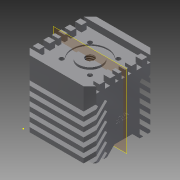
# Autodesk Inventor part: Heatsink
Saved by Autodesk Inventor 2015 (Build 190159000, 159)
## iProperties
Created: 2016-02-25
Part Number: Heatsink
Material: Aluminum 6061-AHC
Document SubType Name: Modeling
Designer: 672301
Density: 2.7 g/cm^3
Appearance: Anodized - Light Gray
Mass: 80.5123 g
Surface Area: 229.153 cm^2
Volume: 29.8194 cm^3
Author: 672301
Autodesk Inventor part; units mm, degrees
(part 1 of 2)
ref_plane "YZ Plane" through (0, 0, 0) normal (1, 0, 0) x (0, 1, 0)
ref_plane "XZ Plane" through (0, 0, 0) normal (0, 1, 0) x (-1, 0, 0)
sketch "Sketch1" plane through (0, 0, 0) normal (0, 1, 0) x (-1, 0, 0)
  line L0 (0, 0) -> (-40.005, 0)
  line L1 (-40.005, 0) -> (-40.005, -40.005)
  line L2 (-40.005, -40.005) -> (0, -40.005)
  line L3 (0, -40.005) -> (0, 0)
  dimension "d0" = 40.005
  dimension "d1" = 40.005
  constraints: 8 end point, 2 parallel, 1 horizontal, 1 perpendicular
  measures "d0" distance of L2.end L1.end
  measures "d1" distance of L0.end L1.end
extrude "Extrusion1" add sketch "Sketch1" along normal blind 40.005
sketch "Sketch2" plane through (0, 40.005, 0) normal (0, 1, 0) x (1, 0, 0)
  line L0 (0, 40.005) -> (0, 0) projected
  line L1 (0, 0) -> (40.005, 0) projected
  line L2 (0, 5.715) -> (40.005, 5.715)
  line L3 (0, 8.89) -> (40.005, 8.89)
  line L4 (0, 12.065) -> (40.005, 12.065)
  line L5 (0, 15.24) -> (40.005, 15.24)
  line L6 (40.005, 0) -> (40.005, 40.005) projected
  line L7 (0, 3.81) -> (40.005, 3.81)
  line L8 (0, 17.145) -> (40.005, 17.145)
  line L9 (0, 19.05) -> (40.005, 19.05)
  line L10 (0, 20.0025) -> (40.005, 20.0025) construction
  line L11 (0, 34.29) -> (40.005, 34.29)
  line L12 (0, 31.115) -> (40.005, 31.115)
  line L13 (0, 27.94) -> (40.005, 27.94)
  line L14 (0, 24.765) -> (40.005, 24.765)
  line L15 (0, 36.195) -> (40.005, 36.195)
  line L16 (0, 22.86) -> (40.005, 22.86)
  line L17 (0, 20.955) -> (40.005, 20.955)
  line L18 (0, 3.81) -> (0, 5.715)
  line L19 (40.005, 3.81) -> (40.005, 5.715)
  line L20 (0, 5.715) -> (0, 8.89)
  line L21 (0, 8.89) -> (0, 12.065)
  line L22 (0, 12.065) -> (0, 15.24)
  line L23 (0, 17.145) -> (0, 15.24)
  line L24 (0, 17.145) -> (0, 19.05)
  line L25 (0, 19.05) -> (0, 20.955)
  line L26 (0, 20.955) -> (0, 22.86)
  line L27 (0, 22.86) -> (0, 24.765)
  line L28 (0, 24.765) -> (0, 27.94)
  line L29 (0, 27.94) -> (0, 31.115)
  line L30 (0, 31.115) -> (0, 34.29)
  line L31 (0, 34.29) -> (0, 36.195)
  line L32 (0, 36.195) -> (0, 40.005)
  line L33 (40.005, 40.005) -> (40.005, 36.195)
  line L34 (40.005, 36.195) -> (40.005, 34.29)
  line L35 (40.005, 34.29) -> (40.005, 31.115)
  line L36 (40.005, 31.115) -> (40.005, 27.94)
  line L37 (40.005, 27.94) -> (40.005, 24.765)
  line L38 (40.005, 24.765) -> (40.005, 22.86)
  line L39 (40.005, 22.86) -> (40.005, 20.955)
  line L40 (40.005, 20.955) -> (40.005, 19.05)
  line L41 (40.005, 19.05) -> (40.005, 17.145)
  line L42 (40.005, 15.24) -> (40.005, 12.065)
  line L43 (40.005, 8.89) -> (40.005, 5.715)
  line L44 (40.005, 5.715) -> (40.005, 3.81)
  line L45 (40.005, 5.715) -> (40.005, 8.89)
  line L46 (0, 3.81) -> (0, 5.715)
  line L47 (40.005, 3.81) -> (40.005, 0)
  line L48 (0, 0) -> (0, 3.81)
  dimension "d5" = 5.715
  dimension "d6" = 8.89
  dimension "d7" = 12.065
  dimension "d8" = 15.24
  dimension "d9" = 3.81
  dimension "d10" = 17.145
  dimension "d11" = 19.05
  constraints: 92 end point, 17 collinear, 14 symmetric about line, 12 vertical, 4 horizontal, 4 point on line, 3 perpendicular, 2 parallel, 1 midpoint, 9 other
  measures "d5" distance between parallel lines of L1 L2
  measures "d6" distance between parallel lines of L1 L3
  measures "d7" distance between parallel lines of L1 L4
  measures "d8" distance between parallel lines of L1 L5
  measures "d9" distance between parallel lines of L1 L7
  measures "d10" distance between parallel lines of L1 L8
  measures "d11" distance between parallel lines of L1 L9
extrude "Extrusion2" cut sketch "Sketch2" against normal blind 3.81 contours L15 L6 L11 L0 | L12 L6 L13 L0 | L14 L6 L16 L0 | L17 L6 L9 L0 | L8 L6 L5 L0 | L4 L6 L3 L0 | L2 L6 L7 L0
sketch "Sketch3" plane through (0, 40.005, 0) normal (0, 1, 0) x (1, 0, 0)
  line L0 (0, 0) -> (0, 3.81)
  line L1 (0, 3.81) -> (3.81, 3.81)
  line L2 (40.005, 3.81) -> (0, 3.81) projected
  line L3 (40.005, 0) -> (40.005, 3.81)
  line L4 (40.005, 3.81) -> (36.195, 3.81)
  line L5 (0, 40.005) -> (0, 36.195)
  line L6 (0, 40.005) -> (0, 36.195) projected
  line L7 (0, 36.195) -> (3.81, 36.195)
  line L8 (0, 36.195) -> (40.005, 36.195) projected
  line L9 (40.005, 40.005) -> (40.005, 36.195)
  line L10 (40.005, 36.195) -> (40.005, 40.005) projected
  line L11 (40.005, 36.195) -> (36.195, 36.195)
  line L12 (3.81, 3.81) -> (36.195, 3.81)
  line L13 (36.195, 3.81) -> (36.195, 36.195)
  line L14 (36.195, 36.195) -> (3.81, 36.195)
  line L15 (3.81, 36.195) -> (3.81, 3.81)
  dimension "d14" = 3.81
  dimension "d15" = 3.81
  dimension "d16" = 3.81
  constraints: 24 end point, 4 equal length, 4 point on line, 2 vertical, 1 horizontal, 1 perpendicular
  measures "d14" distance of L0.start L0.end
  measures "d15" distance of L0.end L1.end
  measures "d16" distance of L2.start L4.end
extrude "Extrusion3" cut sketch "Sketch3" against normal up to surface (3.81 mm away)
sketch "Sketch4" plane through (0, 36.195, 0) normal (0, 1, 0) x (1, 0, 0)
  line L0 (40.005, 40.005) -> (0, 40.005) projected
  line L1 (0, 0) -> (40.005, 0) projected
  line L2 (0, 40.005) -> (0, 0) construction
  line L3 (0, 20.0025) -> (40.005, 20.0025) construction
  line L4 (40.005, 0) -> (40.005, 40.005) construction
  circle A0 centre (20.0025, 20.0025) radius 6.985
  circle A1 centre (20.0025, 20.0025) radius 10.668
  dimension "d19" = 13.97
  dimension "d20" = 21.336
  constraints: 3 midpoint, 2 centre point, 2 end point, 1 coincident
  measures "d19" diameter of A0
  measures "d20" diameter of A1
extrude "Extrusion4" cut sketch "Sketch4" against normal blind 0.762
sketch "Sketch5" plane through (0, 36.195, 0) normal (0, 1, 0) x (1, 0, 0)
  circle A0 centre (20.0025, 20.0025) radius 6.985 projected
  point P0 (0, 0)
extrude "Extrusion5" add sketch "Sketch5" along normal blind 0.508
hole "Hole1" at (20.0025, 36.703, -20.0025) direction (0, -1, 0) diameter 4.9784 end through all thread size "1/4-20 UNC" class "2B" standard "ANSI Unified Screw Threads"
sketch "Sketch6" plane through (0, 36.195, 0) normal (0, 1, 0) x (1, 0, 0)
  circle A0 centre (20.0025, 20.0025) radius 2.4892 projected
  circle A1 centre (20.0025, 20.0025) radius 6.985 projected
  line L0 (28.4861, 28.4861) -> (11.5189, 28.4861) construction
  line L1 (11.5189, 28.4861) -> (11.5189, 11.5189) construction
  line L2 (11.5189, 11.5189) -> (28.4861, 11.5189) construction
  line L3 (28.4861, 11.5189) -> (28.4861, 28.4861) construction
  line L4 (28.4861, 28.4861) -> (11.5189, 11.5189) construction
  line L5 (11.5189, 28.4861) -> (28.4861, 11.5189) construction
  point P0 (0, 0)
  dimension "d34" = 16.9672
  dimension "d35" = 16.9672
  constraints: 12 end point, 2 midpoint, 2 parallel, 1 horizontal, 1 perpendicular
  measures "d34" distance of L2.end L1.end
  measures "d35" distance of L1.end L0.end
hole "Hole2" at (28.4861, 36.195, -28.4861) at (11.5189, 36.195, -28.4861) at (11.5189, 36.195, -11.5189) at (28.4861, 36.195, -11.5189) direction (0, -1, 0) diameter 2.667 end through all
chamfer "Chamfer1" distance 3.81 angle 45 4 edges at (0, 20.0025, -40.005) (0, 20.0025, 0) (40.005, 20.0025, 0) (40.005, 20.0025, -40.005)
sketch "Sketch7" plane through (0, 0, 0) normal (0, -1, 0) x (1, 0, 0)
  line L0 (40.005, -3.81) -> (40.005, -14.605) construction
  line L1 (40.005, -3.81) -> (40.005, -36.195) projected
  line L2 (0, -36.195) -> (0, -3.81) projected
  line L3 (40.005, -14.605) -> (0, -14.605)
  line L4 (0, -14.605) -> (0, -25.4)
  line L5 (0, -25.4) -> (40.005, -25.4)
  line L6 (40.005, -25.4) -> (40.005, -14.605)
  point P0 (0, 0)
  dimension "d46" = 10.795
  dimension "d47" = 10.795
  constraints: 10 end point, 2 parallel, 2 point on line, 1 horizontal, 1 perpendicular
  measures "d46" distance of L0.start L0.end
  measures "d47" distance of L4.end L3.end
extrude "Extrusion6" cut sketch "Sketch7" against normal blind 4.445
sketch "Sketch8" plane through (0, 36.195, -5.715) normal (-1, 0, 0) x (0, 0, 1)
  line L0 (-8.89, -31.75) -> (-4.4778, -36.195)
  line L1 (-8.89, -36.195) -> (1.905, -36.195) projected
  line L2 (-19.685, -31.75) -> (-24.1046, -36.195)
  line L3 (-24.1046, -36.195) -> (-24.1046, 0) projected
  line L4 (-8.89, -31.75) -> (-8.89, -36.195)
  line L5 (-8.89, -31.75) -> (-8.89, -36.195) projected
  line L6 (-19.685, -31.75) -> (-19.685, -36.195)
  line L7 (-19.685, -36.195) -> (-19.685, -31.75) projected
  line L8 (-19.685, -36.195) -> (-24.1046, -36.195)
  line L9 (-30.48, -36.195) -> (-19.685, -36.195) projected
  point P0 (5.715, -36.195)
  constraints: 10 end point, 3 collinear, 2 point on line
extrude "Extrusion7" cut sketch "Sketch8" against normal through all contours L0 L1 L4
sketch "Sketch9" plane through (0, 36.195, -5.715) normal (-1, 0, 0) x (0, 0, 1)
  line L0 (-19.685, -31.75) -> (-24.1159, -36.195)
  line L1 (-30.48, -36.195) -> (-19.685, -36.195) projected
  line L2 (-19.685, -31.75) -> (-19.685, -36.195)
  line L3 (-19.685, -36.195) -> (-24.1159, -36.195)
  point P0 (5.715, -36.195)
  constraints: 6 end point, 1 perpendicular, 1 point on line, 1 vertical
extrude "Extrusion8" cut sketch "Sketch9" against normal through all
sketch "Sketch10" plane through (0, 4.445, 0) normal (0, -1, 0) x (1, 0, 0)
  circle A0 centre (20.0025, -20.0025) radius 2.4892 projected
  line L0 (36.195, -16.8275) -> (3.81, -16.8275)
  line L1 (3.81, -16.8275) -> (3.81, -23.1775)
  line L2 (3.81, -23.1775) -> (36.195, -23.1775)
  line L3 (36.195, -23.1775) -> (36.195, -16.8275)
  line L4 (36.195, -16.8275) -> (3.81, -23.1775) construction
  line L5 (3.81, -16.8275) -> (36.195, -23.1775) construction
  line L6 (40.005, -14.605) -> (40.005, -25.4) projected
  point P0 (0, 0)
  dimension "d54" = 32.385
  dimension "d55" = 6.35
  dimension "d56" = 3.81
  constraints: 12 end point, 2 midpoint, 2 parallel, 1 horizontal, 1 perpendicular
  measures "d54" distance of L2.end L1.end
  measures "d55" distance of L1.end L0.end
  measures "d56" distance between parallel lines of L6 L3
extrude "Extrusion9" cut sketch "Sketch10" against normal blind 16.51
sketch "Sketch12" plane through (36.195, 0, -40.005) normal (0, 0, -1) x (-1, 0, 0)
  point P0 (36.195, 0)
ref_plane "Work Plane1" through (3.81, 20.955, -20.0025) normal (0, 0, 1) x (1, 0, 0)
sketch "Sketch18" plane through (0, 36.195, -5.715) normal (-1, 0, 0) x (0, 0, 1)
  point P0 (5.715, -36.195)
sketch "Sketch19" plane through (0, 36.195, -5.715) normal (-1, 0, 0) x (0, 0, 1)
  point P0 (5.715, -36.195)
sketch "Sketch20" plane through (40.005, 36.195, -34.29) normal (1, 0, 0) x (0, 0, -1)
  line L0 (1.9052, -36.1976) -> (-4.4448, -36.1976)
  line L1 (1.9052, -36.1976) -> (5.7152, -36.1976)
  line L2 (5.7152, -36.1976) -> (5.7152, 3.8074)
  line L3 (5.7152, -36.1976) -> (-4.5592, -25.9231)
  line L4 (3.0212, -36.1976) -> (-4.5592, -28.6172)
  line L5 (0.3271, -36.1976) -> (-4.5592, -31.3113)
  line L6 (5.7152, -33.5035) -> (-4.5592, -23.2291)
  line L7 (-4.5592, -34.0054) -> (-2.367, -36.1976)
  line L8 (-4.5592, -20.535) -> (5.7152, -30.8094)
  line L9 (-4.5592, -17.8409) -> (5.7152, -28.1153)
  line L10 (-4.5592, -15.1468) -> (5.7152, -25.4213)
  line L11 (-4.5592, -12.4528) -> (5.7152, -22.7272)
  line L12 (-4.5592, -9.7587) -> (5.7152, -20.0331)
  line L13 (-4.5592, -7.0646) -> (5.7152, -17.339)
  line L14 (-3.2121, -5.7176) -> (5.7152, -14.645)
  line L15 (0.829, -7.0646) -> (5.7152, -11.9509)
  line L16 (2.176, -5.7176) -> (5.7152, -9.2568)
  line L17 (2.176, -5.7176) -> (0.829, -7.0646)
  line L18 (-3.2121, -5.7176) -> (5.7152, -5.7176)
  line L19 (-3.2121, -5.7176) -> (-4.5592, -7.0646)
  line L20 (-4.5592, -7.0646) -> (-4.5592, -36.0831)
  point P0 (-34.29, -36.195)
  dimension "d99" = 10.2744
  dimension "d85" = 45
  dimension "d86" = 1.905
  dimension "d87" = 3.81
  dimension "d88" = 1.905
  dimension "d89" = 1.905
  dimension "d90" = 1.905
  dimension "d91" = 1.905
  dimension "d92" = 1.905
  dimension "d93" = 1.905
  dimension "d94" = 1.905
  dimension "d95" = 1.905
  dimension "d96" = 1.905
  dimension "d97" = 1.905
  dimension "d98" = 1.905
  constraints: 38 end point, 12 parallel, 4 point on line, 2 horizontal, 2 perpendicular, 27 other
  measures "d85" angle of L0 L3
  measures "d86" distance between parallel lines of L4 L3
  measures "d87" distance between parallel lines of L3 L5
  measures "d88" distance between parallel lines of L3 L6
  measures "d89" distance between parallel lines of L5 L7
  measures "d90" distance between parallel lines of L6 L8
  measures "d91" distance between parallel lines of L8 L9
  measures "d92" distance between parallel lines of L9 L10
  measures "d93" distance between parallel lines of L10 L11
  measures "d94" distance between parallel lines of L11 L12
  measures "d95" distance between parallel lines of L12 L13
  measures "d96" distance between parallel lines of L13 L14
  measures "d97" distance between parallel lines of L14 L15
  measures "d98" distance between parallel lines of L15 L16
extrude "Extrusion14" cut sketch "Sketch20" against normal through all contours L0 L7 L20 L5 | L4 L20 L3 L1 | L6 L20 L8 L2 | L9 L20 L10 L2 | L11 L20 L12 L2 | L13 L19 L14 L2 | L15 L17 L16 L2
mirror "Mirror2" about plane through (3.81, 20.955, -20.0025) normal (0, 0, 1) of "Extrusion14"
sketch "Sketch21" plane through (0, 0, 0) normal (0, 1, 0) x (-1, 0, 0)
  point P0 (0, 0)
sketch "Sketch22" plane through (0, 0, 0) normal (0, -1, 0) x (1, 0, 0)
  arc A0 (11.3789, -10.1928) -> (11.6589, -10.1928) centre (11.5189, -11.5189) ccw projected
  arc A1 (28.3461, -10.1928) -> (28.6261, -10.1928) centre (28.4861, -11.5189) ccw projected
  circle A2 centre (20.0025, -20.0025) radius 2.4892 projected
  circle A3 centre (28.4861, -28.4861) radius 1.3335 projected
  circle A4 centre (11.5189, -28.4861) radius 1.3335 projected
  circle A5 centre (20.0025, -20.0025) radius 11.1125
  circle A6 centre (28.4861, -11.5189) radius 3.175
  circle A7 centre (11.5189, -11.5189) radius 3.175
  circle A8 centre (28.4861, -28.4861) radius 3.175
  circle A9 centre (11.5189, -28.4861) radius 3.175
  line L0 (38.8914, -2.6964) -> (1.1136, -2.6964) projected
  line L1 (0, -3.81) -> (1.1136, -2.6964) projected
  line L2 (0, -5.3905) -> (0, -3.81) projected
  line L3 (0, -5.3905) -> (40.005, -5.3905) projected
  line L4 (40.005, -3.81) -> (40.005, -5.3905) projected
  line L5 (38.8914, -2.6964) -> (40.005, -3.81) projected
  line L6 (40.005, -8.0846) -> (0, -8.0846) projected
  line L7 (0, -10.1928) -> (0, -8.0846) projected
  line L8 (0, -10.1928) -> (11.3789, -10.1928) projected
  arc A10 (11.6589, -10.1928) -> (11.3789, -10.1928) centre (11.5189, -11.5189) ccw projected
  line L9 (11.6589, -10.1928) -> (28.3461, -10.1928) projected
  arc A11 (28.6261, -10.1928) -> (28.3461, -10.1928) centre (28.4861, -11.5189) ccw projected
  line L10 (28.6261, -10.1928) -> (40.005, -10.1928) projected
  line L11 (40.005, -8.0846) -> (40.005, -10.1928) projected
  line L12 (0, -31.9204) -> (40.005, -31.9204) projected
  line L13 (40.005, -29.8309) -> (40.005, -31.9204) projected
  line L14 (40.005, -29.8309) -> (0, -29.8309) projected
  line L15 (0, -31.9204) -> (0, -29.8309) projected
  point P0 (0, 0)
  dimension "d103" = 22.225
  dimension "d105" = 6.35
  dimension "d106" = 6.35
  dimension "d107" = 6.35
  dimension "d108" = 6.35
  constraints: 5 centre point, 5 coincident
  measures "d103" diameter of A5
  measures "d105" diameter of A6
  measures "d106" diameter of A7
  measures "d107" diameter of A8
  measures "d108" diameter of A9
extrude "Extrusion15" cut sketch "Sketch22" against normal blind 31.115 contours A10 A0 A5 | A0 A5 A7 L8 | L8 A7 L9 A10 | A5 A0 | A0 A5 A7 | L9 A7 A5 A0 | A7 A5 L9 A6 A8 L14 A9 | A9 A5 A4 | A5 A4 A9 L14 | A5 L9 | L14 A9 | A6 L9 A1 A5 | A5 A1 A6 | A6 L10 A11 L9 | L14 A5 | A5 A1 | A1 A11 A5 | A5 A1 L10 A6 | A8 A5 A3 | A5 A3 A8 L14 | L14 A8
sketch "Sketch24" plane through (40.005, 4.445, -14.605) normal (1, 0, 0) x (0, 0, -1)
  line L0 (-4.2599, 13.3727) -> (14.146, 13.3727) construction
  line L1 (14.146, 13.3727) -> (14.146, 9.6523) construction
  line L2 (14.146, 9.6523) -> (-4.2599, 9.6523) construction
  line L3 (-4.2599, 9.6523) -> (-4.2599, 13.3727) construction
  spline S0 degree 2 poles (3.1149, 12.9571) (3.1149, 12.8527) (3.0303, 12.6848) (2.9593, 12.6378) knots 0 0 0 1 2 2 2
  spline S1 degree 2 poles (2.9593, 12.6378) (2.9013, 12.6014) (2.7821, 12.5767) (2.6895, 12.5767) knots 0 0 0 1 2 2 2
  line L4 (2.6895, 12.5767) -> (2.5141, 12.5767)
  line L5 (2.5141, 12.5767) -> (2.5141, 13.3387)
  line L6 (2.5141, 13.3387) -> (2.6876, 13.3387)
  spline S2 degree 2 poles (2.6876, 13.3387) (2.7951, 13.3387) (2.9173, 13.3066) (2.9606, 13.2782) knots 0 0 0 1 2 2 2
  spline S3 degree 2 poles (2.9606, 13.2782) (3.034, 13.2294) (3.1149, 13.0682) (3.1149, 12.9571) knots 0 0 0 1 2 2 2
  spline S4 degree 2 poles (3.0093, 12.9583) (3.0093, 13.046) (2.9513, 13.1701) (2.8939, 13.2053) knots 0 0 0 1 2 2 2
  spline S5 degree 2 poles (2.8939, 13.2053) (2.8531, 13.2294) (2.7611, 13.251) (2.6926, 13.251) knots 0 0 0 1 2 2 2
  line L7 (2.6926, 13.251) -> (2.6154, 13.251)
  line L8 (2.6154, 13.251) -> (2.6154, 12.6644)
  line L9 (2.6154, 12.6644) -> (2.6926, 12.6644)
  spline S6 degree 2 poles (2.6926, 12.6644) (2.7599, 12.6644) (2.8618, 12.686) (2.9031, 12.715) knots 0 0 0 1 2 2 2
  spline S7 degree 2 poles (2.9031, 12.715) (2.9562, 12.7508) (3.0093, 12.8694) (3.0093, 12.9583) knots 0 0 0 1 2 2 2
  spline S8 degree 2 poles (3.5361, 12.6372) (3.5243, 12.6286) (3.4848, 12.5977) (3.4663, 12.5884) knots 0 0 0 1 2 2 2
  spline S9 degree 2 poles (3.4663, 12.5884) (3.441, 12.5749) (3.3934, 12.5607) (3.3502, 12.5607) knots 0 0 0 1 2 2 2
  spline S10 degree 2 poles (3.3502, 12.5607) (3.315, 12.5607) (3.2514, 12.5872) (3.2273, 12.6113) knots 0 0 0 1 2 2 2
  spline S11 degree 2 poles (3.2273, 12.6113) (3.2045, 12.6348) (3.1767, 12.7039) (3.1767, 12.7422) knots 0 0 0 1 2 2 2
  spline S12 degree 2 poles (3.1767, 12.7422) (3.1767, 12.8015) (3.2267, 12.8855) (3.281, 12.9095) knots 0 0 0 1 2 2 2
  spline S13 degree 2 poles (3.281, 12.9095) (3.3292, 12.9318) (3.4601, 12.9485) (3.5361, 12.9528) knots 0 0 0 1 2 2 2
  line L10 (3.5361, 12.9528) -> (3.5361, 12.9713)
  spline S14 degree 2 poles (3.5361, 12.9713) (3.5361, 13.0046) (3.5157, 13.046) (3.4972, 13.0577) knots 0 0 0 1 2 2 2
  spline S15 degree 2 poles (3.4972, 13.0577) (3.4786, 13.0695) (3.4255, 13.0769) (3.3971, 13.0769) knots 0 0 0 1 2 2 2
  spline S16 degree 2 poles (3.3971, 13.0769) (3.3638, 13.0769) (3.2736, 13.0571) (3.2285, 13.038) knots 0 0 0 1 2 2 2
  line L11 (3.2285, 13.038) -> (3.223, 13.038)
  line L12 (3.223, 13.038) -> (3.223, 13.1362)
  spline S17 degree 2 poles (3.223, 13.1362) (3.2495, 13.1436) (3.349, 13.1621) (3.3977, 13.1621) knots 0 0 0 1 2 2 2
  spline S18 degree 2 poles (3.3977, 13.1621) (3.457, 13.1621) (3.5379, 13.1436) (3.57, 13.1195) knots 0 0 0 1 2 2 2
  spline S19 degree 2 poles (3.57, 13.1195) (3.6015, 13.096) (3.6324, 13.0213) (3.6324, 12.9676) knots 0 0 0 1 2 2 2
  line L13 (3.6324, 12.9676) -> (3.6324, 12.5767)
  line L14 (3.6324, 12.5767) -> (3.5361, 12.5767)
  line L15 (3.5361, 12.5767) -> (3.5361, 12.6372)
  line L16 (3.5361, 12.7175) -> (3.5361, 12.8762)
  spline S20 degree 2 poles (3.5361, 12.8762) (3.5015, 12.8731) (3.3971, 12.8626) (3.3644, 12.8527) knots 0 0 0 1 2 2 2
  spline S21 degree 2 poles (3.3644, 12.8527) (3.3261, 12.841) (3.2761, 12.7922) (3.2761, 12.749) knots 0 0 0 1 2 2 2
  spline S22 degree 2 poles (3.2761, 12.749) (3.2761, 12.6996) (3.3317, 12.6496) (3.3848, 12.6496) knots 0 0 0 1 2 2 2
  spline S23 degree 2 poles (3.3848, 12.6496) (3.4299, 12.6496) (3.504, 12.6885) (3.5361, 12.7175) knots 0 0 0 1 2 2 2
  line L17 (4.0708, 13.0454) -> (4.0659, 13.0454)
  spline S24 degree 2 poles (4.0659, 13.0454) (4.0548, 13.0485) (4.0307, 13.0497) (4.014, 13.0497) knots 0 0 0 1 2 2 2
  spline S25 degree 2 poles (4.014, 13.0497) (3.9751, 13.0497) (3.8985, 13.0158) (3.864, 12.9824) knots 0 0 0 1 2 2 2
  line L18 (3.864, 12.9824) -> (3.864, 12.5767)
  line L19 (3.864, 12.5767) -> (3.7676, 12.5767)
  line L20 (3.7676, 12.5767) -> (3.7676, 13.1485)
  line L21 (3.7676, 13.1485) -> (3.864, 13.1485)
  line L22 (3.864, 13.1485) -> (3.864, 13.0633)
  spline S26 degree 2 poles (3.864, 13.0633) (3.9164, 13.1102) (3.9949, 13.1485) (4.0319, 13.1485) knots 0 0 0 1 2 2 2
  spline S27 degree 2 poles (4.0319, 13.1485) (4.0467, 13.1485) (4.0616, 13.1473) (4.0708, 13.1454) knots 0 0 0 1 2 2 2
  line L23 (4.0708, 13.1454) -> (4.0708, 13.0454)
  spline S28 degree 2 poles (4.2999, 12.5631) (4.2425, 12.5631) (4.1431, 12.594) (4.1103, 12.6113) knots 0 0 0 1 2 2 2
  line L24 (4.1103, 12.6113) -> (4.1103, 12.7194)
  line L25 (4.1103, 12.7194) -> (4.1153, 12.7194)
  spline S29 degree 2 poles (4.1153, 12.7194) (4.1276, 12.7095) (4.161, 12.686) (4.1888, 12.673) knots 0 0 0 1 2 2 2
  spline S30 degree 2 poles (4.1888, 12.673) (4.2129, 12.6613) (4.2721, 12.644) (4.3036, 12.644) knots 0 0 0 1 2 2 2
  spline S31 degree 2 poles (4.3036, 12.644) (4.3265, 12.644) (4.379, 12.6545) (4.3913, 12.6632) knots 0 0 0 1 2 2 2
  spline S32 degree 2 poles (4.3913, 12.6632) (4.4092, 12.6749) (4.4253, 12.7014) (4.4253, 12.7286) knots 0 0 0 1 2 2 2
  spline S33 degree 2 poles (4.4253, 12.7286) (4.4253, 12.7626) (4.3882, 12.7978) (4.3407, 12.8095) knots 0 0 0 1 2 2 2
  spline S34 degree 2 poles (4.3407, 12.8095) (4.3221, 12.8138) (4.2629, 12.8262) (4.2376, 12.833) knots 0 0 0 1 2 2 2
  spline S35 degree 2 poles (4.2376, 12.833) (4.1721, 12.8521) (4.1128, 12.9312) (4.1128, 12.9874) knots 0 0 0 1 2 2 2
  spline S36 degree 2 poles (4.1128, 12.9874) (4.1128, 13.0652) (4.2295, 13.1621) (4.3259, 13.1621) knots 0 0 0 1 2 2 2
  spline S37 degree 2 poles (4.3259, 13.1621) (4.3734, 13.1621) (4.4697, 13.1386) (4.5025, 13.1207) knots 0 0 0 1 2 2 2
  line L26 (4.5025, 13.1207) -> (4.5025, 13.0176)
  line L27 (4.5025, 13.0176) -> (4.4975, 13.0176)
  spline S38 degree 2 poles (4.4975, 13.0176) (4.4605, 13.0473) (4.3703, 13.0812) (4.324, 13.0812) knots 0 0 0 1 2 2 2
  spline S39 degree 2 poles (4.324, 13.0812) (4.2765, 13.0812) (4.211, 13.0411) (4.211, 13.0009) knots 0 0 0 1 2 2 2
  spline S40 degree 2 poles (4.211, 13.0009) (4.211, 12.9645) (4.2499, 12.9293) (4.2931, 12.9182) knots 0 0 0 1 2 2 2
  spline S41 degree 2 poles (4.2931, 12.9182) (4.3141, 12.9126) (4.3672, 12.9015) (4.3962, 12.8947) knots 0 0 0 1 2 2 2
  spline S42 degree 2 poles (4.3962, 12.8947) (4.4592, 12.8787) (4.5235, 12.8052) (4.5235, 12.7416) knots 0 0 0 1 2 2 2
  spline S43 degree 2 poles (4.5235, 12.7416) (4.5235, 12.7045) (4.4944, 12.6391) (4.466, 12.615) knots 0 0 0 1 2 2 2
  spline S44 degree 2 poles (4.466, 12.615) (4.4358, 12.5897) (4.3586, 12.5631) (4.2999, 12.5631) knots 0 0 0 1 2 2 2
  line L28 (5.0619, 12.5767) -> (4.9656, 12.5767)
  line L29 (4.9656, 12.5767) -> (4.9656, 12.9028)
  spline S45 degree 2 poles (4.9656, 12.9028) (4.9656, 12.9423) (4.9582, 13.0102) (4.9471, 13.0306) knots 0 0 0 1 2 2 2
  spline S46 degree 2 poles (4.9471, 13.0306) (4.9353, 13.0522) (4.8933, 13.0732) (4.8575, 13.0732) knots 0 0 0 1 2 2 2
  spline S47 degree 2 poles (4.8575, 13.0732) (4.8217, 13.0732) (4.7458, 13.0349) (4.7093, 13.004) knots 0 0 0 1 2 2 2
  line L30 (4.7093, 13.004) -> (4.7093, 12.5767)
  line L31 (4.7093, 12.5767) -> (4.613, 12.5767)
  line L32 (4.613, 12.5767) -> (4.613, 13.3727)
  line L33 (4.613, 13.3727) -> (4.7093, 13.3727)
  line L34 (4.7093, 13.3727) -> (4.7093, 13.0849)
  spline S48 degree 2 poles (4.7093, 13.0849) (4.7525, 13.1238) (4.8359, 13.1646) (4.8828, 13.1646) knots 0 0 0 1 2 2 2
  spline S49 degree 2 poles (4.8828, 13.1646) (4.9668, 13.1646) (5.0619, 13.0534) (5.0619, 12.9478) knots 0 0 0 1 2 2 2
  line L35 (5.0619, 12.9478) -> (5.0619, 12.5767)
  line L36 (5.2953, 12.5767) -> (5.199, 12.5767)
  line L37 (5.199, 12.5767) -> (5.199, 13.1485)
  line L38 (5.199, 13.1485) -> (5.2953, 13.1485)
  line L39 (5.2953, 13.1485) -> (5.2953, 12.5767)
  line L40 (5.3021, 13.2436) -> (5.1928, 13.2436)
  line L41 (5.1928, 13.2436) -> (5.1928, 13.3437)
  line L42 (5.1928, 13.3437) -> (5.3021, 13.3437)
  line L43 (5.3021, 13.3437) -> (5.3021, 13.2436)
  line L44 (5.5349, 12.5767) -> (5.4386, 12.5767)
  line L45 (5.4386, 12.5767) -> (5.4386, 13.3727)
  line L46 (5.4386, 13.3727) -> (5.5349, 13.3727)
  line L47 (5.5349, 13.3727) -> (5.5349, 12.5767)
  spline S50 degree 2 poles (6.3087, 12.5631) (6.2346, 12.5631) (6.1092, 12.6131) (6.0635, 12.6632) knots 0 0 0 1 2 2 2
  spline S51 degree 2 poles (6.0635, 12.6632) (6.0178, 12.7126) (5.9678, 12.8608) (5.9678, 12.9571) knots 0 0 0 1 2 2 2
  spline S52 degree 2 poles (5.9678, 12.9571) (5.9678, 13.0528) (6.0166, 13.1948) (6.0629, 13.2473) knots 0 0 0 1 2 2 2
  spline S53 degree 2 poles (6.0629, 13.2473) (6.1086, 13.2986) (6.2333, 13.3523) (6.3105, 13.3523) knots 0 0 0 1 2 2 2
  spline S54 degree 2 poles (6.3105, 13.3523) (6.3488, 13.3523) (6.4161, 13.3412) (6.4445, 13.3325) knots 0 0 0 1 2 2 2
  spline S55 degree 2 poles (6.4445, 13.3325) (6.4692, 13.3245) (6.5205, 13.3017) (6.5458, 13.2881) knots 0 0 0 1 2 2 2
  line L48 (6.5458, 13.2881) -> (6.5458, 13.1658)
  line L49 (6.5458, 13.1658) -> (6.5378, 13.1658)
  spline S56 degree 2 poles (6.5378, 13.1658) (6.5242, 13.1782) (6.4822, 13.2127) (6.4519, 13.2294) knots 0 0 0 1 2 2 2
  spline S57 degree 2 poles (6.4519, 13.2294) (6.4229, 13.2455) (6.3544, 13.2658) (6.3099, 13.2658) knots 0 0 0 1 2 2 2
  spline S58 degree 2 poles (6.3099, 13.2658) (6.2611, 13.2658) (6.174, 13.2257) (6.1413, 13.1874) knots 0 0 0 1 2 2 2
  spline S59 degree 2 poles (6.1413, 13.1874) (6.1092, 13.1485) (6.0734, 13.0306) (6.0734, 12.9571) knots 0 0 0 1 2 2 2
  spline S60 degree 2 poles (6.0734, 12.9571) (6.0734, 12.8787) (6.1111, 12.7657) (6.1438, 12.7268) knots 0 0 0 1 2 2 2
  spline S61 degree 2 poles (6.1438, 12.7268) (6.1759, 12.6891) (6.2617, 12.6508) (6.3099, 12.6508) knots 0 0 0 1 2 2 2
  spline S62 degree 2 poles (6.3099, 12.6508) (6.3537, 12.6508) (6.4285, 12.6724) (6.4575, 12.6885) knots 0 0 0 1 2 2 2
  spline S63 degree 2 poles (6.4575, 12.6885) (6.4853, 12.7045) (6.5266, 12.7379) (6.5384, 12.7496) knots 0 0 0 1 2 2 2
  line L50 (6.5384, 12.7496) -> (6.5458, 12.7496)
  line L51 (6.5458, 12.7496) -> (6.5458, 12.6286)
  spline S64 degree 2 poles (6.5458, 12.6286) (6.5205, 12.6169) (6.476, 12.5952) (6.4445, 12.5854) knots 0 0 0 1 2 2 2
  spline S65 degree 2 poles (6.4445, 12.5854) (6.4112, 12.5742) (6.3544, 12.5631) (6.3087, 12.5631) knots 0 0 0 1 2 2 2
  spline S66 degree 2 poles (7.1028, 12.8626) (7.1028, 12.7181) (6.9638, 12.5607) (6.8477, 12.5607) knots 0 0 0 1 2 2 2
  spline S67 degree 2 poles (6.8477, 12.5607) (6.7286, 12.5607) (6.5921, 12.7231) (6.5921, 12.8626) knots 0 0 0 1 2 2 2
  spline S68 degree 2 poles (6.5921, 12.8626) (6.5921, 13.0059) (6.7329, 13.1646) (6.8477, 13.1646) knots 0 0 0 1 2 2 2
  spline S69 degree 2 poles (6.8477, 13.1646) (6.9638, 13.1646) (7.1028, 13.0065) (7.1028, 12.8626) knots 0 0 0 1 2 2 2
  spline S70 degree 2 poles (7.0034, 12.8626) (7.0034, 12.9738) (6.9225, 13.0818) (6.8477, 13.0818) knots 0 0 0 1 2 2 2
  spline S71 degree 2 poles (6.8477, 13.0818) (6.773, 13.0818) (6.6915, 12.9738) (6.6915, 12.8626) knots 0 0 0 1 2 2 2
  spline S72 degree 2 poles (6.6915, 12.8626) (6.6915, 12.7546) (6.773, 12.6434) (6.8477, 12.6434) knots 0 0 0 1 2 2 2
  spline S73 degree 2 poles (6.8477, 12.6434) (6.9218, 12.6434) (7.0034, 12.7527) (7.0034, 12.8626) knots 0 0 0 1 2 2 2
  line L52 (7.351, 12.5767) -> (7.2287, 12.5767)
  line L53 (7.2287, 12.5767) -> (7.2287, 12.7224)
  line L54 (7.2287, 12.7224) -> (7.351, 12.7224)
  line L55 (7.351, 12.7224) -> (7.351, 12.5767)
  spline S74 degree 2 poles (1.452, 11.8544) (1.452, 11.805) (1.4168, 11.7161) (1.3853, 11.6852) knots 0 0 0 1 2 2 2
  spline S75 degree 2 poles (1.3853, 11.6852) (1.3458, 11.6463) (1.239, 11.6062) (1.1574, 11.6062) knots 0 0 0 1 2 2 2
  line L56 (1.1574, 11.6062) -> (1.0716, 11.6062)
  line L57 (1.0716, 11.6062) -> (1.0716, 11.3221)
  line L58 (1.0716, 11.3221) -> (0.9703, 11.3221)
  line L59 (0.9703, 11.3221) -> (0.9703, 12.0841)
  line L60 (0.9703, 12.0841) -> (1.1618, 12.0841)
  spline S76 degree 2 poles (1.1618, 12.0841) (1.2297, 12.0841) (1.3248, 12.0619) (1.3612, 12.0366) knots 0 0 0 1 2 2 2
  spline S77 degree 2 poles (1.3612, 12.0366) (1.4038, 12.0075) (1.452, 11.918) (1.452, 11.8544) knots 0 0 0 1 2 2 2
  spline S78 degree 2 poles (1.3464, 11.8513) (1.3464, 11.8908) (1.3192, 11.9489) (1.2914, 11.9674) knots 0 0 0 1 2 2 2
  spline S79 degree 2 poles (1.2914, 11.9674) (1.2674, 11.9834) (1.2031, 11.9964) (1.1556, 11.9964) knots 0 0 0 1 2 2 2
  line L61 (1.1556, 11.9964) -> (1.0716, 11.9964)
  line L62 (1.0716, 11.9964) -> (1.0716, 11.6926)
  line L63 (1.0716, 11.6926) -> (1.1408, 11.6926)
  spline S80 degree 2 poles (1.1408, 11.6926) (1.2025, 11.6926) (1.2785, 11.7124) (1.3032, 11.7383) knots 0 0 0 1 2 2 2
  spline S81 degree 2 poles (1.3032, 11.7383) (1.326, 11.7611) (1.3464, 11.8149) (1.3464, 11.8513) knots 0 0 0 1 2 2 2
  spline S82 degree 2 poles (1.8595, 11.3826) (1.8478, 11.374) (1.8083, 11.3431) (1.7898, 11.3338) knots 0 0 0 1 2 2 2
  spline S83 degree 2 poles (1.7898, 11.3338) (1.7644, 11.3202) (1.7169, 11.306) (1.6737, 11.306) knots 0 0 0 1 2 2 2
  spline S84 degree 2 poles (1.6737, 11.306) (1.6385, 11.306) (1.5749, 11.3326) (1.5508, 11.3567) knots 0 0 0 1 2 2 2
  spline S85 degree 2 poles (1.5508, 11.3567) (1.5279, 11.3801) (1.5002, 11.4493) (1.5002, 11.4876) knots 0 0 0 1 2 2 2
  spline S86 degree 2 poles (1.5002, 11.4876) (1.5002, 11.5469) (1.5502, 11.6309) (1.6045, 11.6549) knots 0 0 0 1 2 2 2
  spline S87 degree 2 poles (1.6045, 11.6549) (1.6527, 11.6772) (1.7836, 11.6938) (1.8595, 11.6982) knots 0 0 0 1 2 2 2
  line L64 (1.8595, 11.6982) -> (1.8595, 11.7167)
  spline S88 degree 2 poles (1.8595, 11.7167) (1.8595, 11.75) (1.8392, 11.7914) (1.8206, 11.8031) knots 0 0 0 1 2 2 2
  spline S89 degree 2 poles (1.8206, 11.8031) (1.8021, 11.8149) (1.749, 11.8223) (1.7206, 11.8223) knots 0 0 0 1 2 2 2
  spline S90 degree 2 poles (1.7206, 11.8223) (1.6873, 11.8223) (1.5971, 11.8025) (1.552, 11.7834) knots 0 0 0 1 2 2 2
  line L65 (1.552, 11.7834) -> (1.5465, 11.7834)
  line L66 (1.5465, 11.7834) -> (1.5465, 11.8816)
  spline S91 degree 2 poles (1.5465, 11.8816) (1.573, 11.889) (1.6724, 11.9075) (1.7212, 11.9075) knots 0 0 0 1 2 2 2
  spline S92 degree 2 poles (1.7212, 11.9075) (1.7805, 11.9075) (1.8614, 11.889) (1.8935, 11.8649) knots 0 0 0 1 2 2 2
  spline S93 degree 2 poles (1.8935, 11.8649) (1.925, 11.8414) (1.9559, 11.7667) (1.9559, 11.713) knots 0 0 0 1 2 2 2
  line L67 (1.9559, 11.713) -> (1.9559, 11.3221)
  line L68 (1.9559, 11.3221) -> (1.8595, 11.3221)
  line L69 (1.8595, 11.3221) -> (1.8595, 11.3826)
  line L70 (1.8595, 11.4629) -> (1.8595, 11.6216)
  spline S94 degree 2 poles (1.8595, 11.6216) (1.825, 11.6185) (1.7206, 11.608) (1.6879, 11.5981) knots 0 0 0 1 2 2 2
  spline S95 degree 2 poles (1.6879, 11.5981) (1.6496, 11.5864) (1.5996, 11.5376) (1.5996, 11.4944) knots 0 0 0 1 2 2 2
  spline S96 degree 2 poles (1.5996, 11.4944) (1.5996, 11.445) (1.6551, 11.395) (1.7083, 11.395) knots 0 0 0 1 2 2 2
  spline S97 degree 2 poles (1.7083, 11.395) (1.7533, 11.395) (1.8274, 11.4339) (1.8595, 11.4629) knots 0 0 0 1 2 2 2
  line L71 (2.3943, 11.7908) -> (2.3894, 11.7908)
  spline S98 degree 2 poles (2.3894, 11.7908) (2.3782, 11.7939) (2.3542, 11.7951) (2.3375, 11.7951) knots 0 0 0 1 2 2 2
  spline S99 degree 2 poles (2.3375, 11.7951) (2.2986, 11.7951) (2.222, 11.7611) (2.1874, 11.7278) knots 0 0 0 1 2 2 2
  line L72 (2.1874, 11.7278) -> (2.1874, 11.3221)
  line L73 (2.1874, 11.3221) -> (2.0911, 11.3221)
  line L74 (2.0911, 11.3221) -> (2.0911, 11.8939)
  line L75 (2.0911, 11.8939) -> (2.1874, 11.8939)
  line L76 (2.1874, 11.8939) -> (2.1874, 11.8087)
  spline S100 degree 2 poles (2.1874, 11.8087) (2.2399, 11.8556) (2.3183, 11.8939) (2.3554, 11.8939) knots 0 0 0 1 2 2 2
  spline S101 degree 2 poles (2.3554, 11.8939) (2.3702, 11.8939) (2.385, 11.8927) (2.3943, 11.8908) knots 0 0 0 1 2 2 2
  line L77 (2.3943, 11.8908) -> (2.3943, 11.7908)
  spline S102 degree 2 poles (2.6419, 11.311) (2.5635, 11.311) (2.4752, 11.4005) (2.4752, 11.4975) knots 0 0 0 1 2 2 2
  line L78 (2.4752, 11.4975) -> (2.4752, 11.8143)
  line L79 (2.4752, 11.8143) -> (2.4104, 11.8143)
  line L80 (2.4104, 11.8143) -> (2.4104, 11.8939)
  line L81 (2.4104, 11.8939) -> (2.4752, 11.8939)
  line L82 (2.4752, 11.8939) -> (2.4752, 12.0582)
  line L83 (2.4752, 12.0582) -> (2.5715, 12.0582)
  line L84 (2.5715, 12.0582) -> (2.5715, 11.8939)
  line L85 (2.5715, 11.8939) -> (2.7487, 11.8939)
  line L86 (2.7487, 11.8939) -> (2.7487, 11.8143)
  line L87 (2.7487, 11.8143) -> (2.5715, 11.8143)
  line L88 (2.5715, 11.8143) -> (2.5715, 11.5419)
  spline S103 degree 2 poles (2.5715, 11.5419) (2.5715, 11.4987) (2.5746, 11.4512) (2.5851, 11.4308) knots 0 0 0 1 2 2 2
  spline S104 degree 2 poles (2.5851, 11.4308) (2.5938, 11.4129) (2.6327, 11.395) (2.666, 11.395) knots 0 0 0 1 2 2 2
  spline S105 degree 2 poles (2.666, 11.395) (2.6895, 11.395) (2.7333, 11.4092) (2.7432, 11.4135) knots 0 0 0 1 2 2 2
  line L89 (2.7432, 11.4135) -> (2.7487, 11.4135)
  line L90 (2.7487, 11.4135) -> (2.7487, 11.327)
  spline S106 degree 2 poles (2.7487, 11.327) (2.7216, 11.3196) (2.666, 11.311) (2.6419, 11.311) knots 0 0 0 1 2 2 2
  line L91 (3.6997, 11.3221) -> (3.5861, 11.3221)
  line L92 (3.5861, 11.3221) -> (3.2489, 11.9791)
  line L93 (3.2489, 11.9791) -> (3.2489, 11.3221)
  line L94 (3.2489, 11.3221) -> (3.1544, 11.3221)
  line L95 (3.1544, 11.3221) -> (3.1544, 12.0841)
  line L96 (3.1544, 12.0841) -> (3.2983, 12.0841)
  line L97 (3.2983, 12.0841) -> (3.6052, 11.4808)
  line L98 (3.6052, 11.4808) -> (3.6052, 12.0841)
  line L99 (3.6052, 12.0841) -> (3.6997, 12.0841)
  line L100 (3.6997, 12.0841) -> (3.6997, 11.3221)
  spline S107 degree 2 poles (4.3166, 11.608) (4.3166, 11.4635) (4.1777, 11.306) (4.0616, 11.306) knots 0 0 0 1 2 2 2
  spline S108 degree 2 poles (4.0616, 11.306) (3.9424, 11.306) (3.8059, 11.4684) (3.8059, 11.608) knots 0 0 0 1 2 2 2
  spline S109 degree 2 poles (3.8059, 11.608) (3.8059, 11.7513) (3.9467, 11.91) (4.0616, 11.91) knots 0 0 0 1 2 2 2
  spline S110 degree 2 poles (4.0616, 11.91) (4.1777, 11.91) (4.3166, 11.7519) (4.3166, 11.608) knots 0 0 0 1 2 2 2
  spline S111 degree 2 poles (4.2172, 11.608) (4.2172, 11.7192) (4.1363, 11.8272) (4.0616, 11.8272) knots 0 0 0 1 2 2 2
  spline S112 degree 2 poles (4.0616, 11.8272) (3.9868, 11.8272) (3.9053, 11.7192) (3.9053, 11.608) knots 0 0 0 1 2 2 2
  spline S113 degree 2 poles (3.9053, 11.608) (3.9053, 11.4999) (3.9868, 11.3888) (4.0616, 11.3888) knots 0 0 0 1 2 2 2
  spline S114 degree 2 poles (4.0616, 11.3888) (4.1357, 11.3888) (4.2172, 11.4981) (4.2172, 11.608) knots 0 0 0 1 2 2 2
  line L101 (4.5648, 11.3221) -> (4.4426, 11.3221)
  line L102 (4.4426, 11.3221) -> (4.4426, 11.4678)
  line L103 (4.4426, 11.4678) -> (4.5648, 11.4678)
  line L104 (4.5648, 11.4678) -> (4.5648, 11.3221)
  line L105 (5.5158, 11.3221) -> (5.0459, 11.3221)
  line L106 (5.0459, 11.3221) -> (5.0459, 11.4302)
  spline S115 degree 2 poles (5.0459, 11.4302) (5.0965, 11.4777) (5.1867, 11.566) (5.2299, 11.6136) knots 0 0 0 1 2 2 2
  spline S116 degree 2 poles (5.2299, 11.6136) (5.3169, 11.7093) (5.3806, 11.8241) (5.3806, 11.8853) knots 0 0 0 1 2 2 2
  spline S117 degree 2 poles (5.3806, 11.8853) (5.3806, 11.9174) (5.3608, 11.9655) (5.3429, 11.981) knots 0 0 0 1 2 2 2
  spline S118 degree 2 poles (5.3429, 11.981) (5.325, 11.9964) (5.278, 12.0119) (5.2496, 12.0119) knots 0 0 0 1 2 2 2
  spline S119 degree 2 poles (5.2496, 12.0119) (5.2225, 12.0119) (5.1669, 11.9983) (5.1416, 11.9878) knots 0 0 0 1 2 2 2
  spline S120 degree 2 poles (5.1416, 11.9878) (5.12, 11.9791) (5.0798, 11.9544) (5.0675, 11.9458) knots 0 0 0 1 2 2 2
  line L107 (5.0675, 11.9458) -> (5.0619, 11.9458)
  line L108 (5.0619, 11.9458) -> (5.0619, 12.0545)
  spline S121 degree 2 poles (5.0619, 12.0545) (5.0934, 12.0699) (5.2064, 12.1002) (5.2571, 12.1002) knots 0 0 0 1 2 2 2
  spline S122 degree 2 poles (5.2571, 12.1002) (5.3639, 12.1002) (5.4843, 11.9872) (5.4843, 11.8908) knots 0 0 0 1 2 2 2
  spline S123 degree 2 poles (5.4843, 11.8908) (5.4843, 11.8457) (5.4633, 11.7704) (5.4448, 11.7383) knots 0 0 0 1 2 2 2
  spline S124 degree 2 poles (5.4448, 11.7383) (5.4262, 11.705) (5.3725, 11.6395) (5.3429, 11.608) knots 0 0 0 1 2 2 2
  spline S125 degree 2 poles (5.3429, 11.608) (5.2947, 11.5555) (5.1768, 11.4431) (5.1416, 11.4104) knots 0 0 0 1 2 2 2
  line L109 (5.1416, 11.4104) -> (5.5158, 11.4104)
  line L110 (5.5158, 11.4104) -> (5.5158, 11.3221)
  line L111 (6.108, 11.5839) -> (6.0172, 11.5839)
  line L112 (6.0172, 11.5839) -> (6.0172, 11.3221)
  line L113 (6.0172, 11.3221) -> (5.919, 11.3221)
  line L114 (5.919, 11.3221) -> (5.919, 11.5839)
  line L115 (5.919, 11.5839) -> (5.5825, 11.5839)
  line L116 (5.5825, 11.5839) -> (5.5825, 11.6914)
  line L117 (5.5825, 11.6914) -> (5.9233, 12.0841)
  line L118 (5.9233, 12.0841) -> (6.0172, 12.0841)
  line L119 (6.0172, 12.0841) -> (6.0172, 11.6661)
  line L120 (6.0172, 11.6661) -> (6.108, 11.6661)
  line L121 (6.108, 11.6661) -> (6.108, 11.5839)
  line L122 (5.919, 11.6661) -> (5.919, 11.9637)
  line L123 (5.919, 11.9637) -> (5.6628, 11.6661)
  line L124 (5.6628, 11.6661) -> (5.919, 11.6661)
  spline S126 degree 2 poles (6.6514, 11.5642) (6.6514, 11.5092) (6.6162, 11.4153) (6.5841, 11.3808) knots 0 0 0 1 2 2 2
  spline S127 degree 2 poles (6.5841, 11.3808) (6.552, 11.3462) (6.4562, 11.306) (6.397, 11.306) knots 0 0 0 1 2 2 2
  spline S128 degree 2 poles (6.397, 11.306) (6.3426, 11.306) (6.2364, 11.3301) (6.1975, 11.3493) knots 0 0 0 1 2 2 2
  line L125 (6.1975, 11.3493) -> (6.1975, 11.4573)
  line L126 (6.1975, 11.4573) -> (6.2049, 11.4573)
  spline S129 degree 2 poles (6.2049, 11.4573) (6.2167, 11.4487) (6.2605, 11.4265) (6.287, 11.4166) knots 0 0 0 1 2 2 2
  spline S130 degree 2 poles (6.287, 11.4166) (6.3173, 11.4061) (6.3673, 11.3943) (6.3988, 11.3943) knots 0 0 0 1 2 2 2
  spline S131 degree 2 poles (6.3988, 11.3943) (6.4297, 11.3943) (6.4877, 11.4166) (6.5087, 11.4407) knots 0 0 0 1 2 2 2
  spline S132 degree 2 poles (6.5087, 11.4407) (6.5279, 11.4635) (6.5476, 11.524) (6.5476, 11.5648) knots 0 0 0 1 2 2 2
  spline S133 degree 2 poles (6.5476, 11.5648) (6.5476, 11.6055) (6.5254, 11.6574) (6.5044, 11.6747) knots 0 0 0 1 2 2 2
  spline S134 degree 2 poles (6.5044, 11.6747) (6.4828, 11.6938) (6.4186, 11.7099) (6.3797, 11.7099) knots 0 0 0 1 2 2 2
  spline S135 degree 2 poles (6.3797, 11.7099) (6.3377, 11.7099) (6.2543, 11.6969) (6.229, 11.6914) knots 0 0 0 1 2 2 2
  line L127 (6.229, 11.6914) -> (6.229, 12.0841)
  line L128 (6.229, 12.0841) -> (6.6471, 12.0841)
  line L129 (6.6471, 12.0841) -> (6.6471, 11.9946)
  line L130 (6.6471, 11.9946) -> (6.3272, 11.9946)
  line L131 (6.3272, 11.9946) -> (6.3272, 11.7914)
  spline S136 degree 2 poles (6.3272, 11.7914) (6.3457, 11.7939) (6.3815, 11.7957) (6.3963, 11.7957) knots 0 0 0 1 2 2 2
  spline S137 degree 2 poles (6.3963, 11.7957) (6.455, 11.7957) (6.5359, 11.7766) (6.573, 11.7482) knots 0 0 0 1 2 2 2
  spline S138 degree 2 poles (6.573, 11.7482) (6.6106, 11.7198) (6.6514, 11.6333) (6.6514, 11.5642) knots 0 0 0 1 2 2 2
  spline S139 degree 2 poles (7.2429, 11.5691) (7.2429, 11.5104) (7.204, 11.411) (7.1713, 11.3777) knots 0 0 0 1 2 2 2
  spline S140 degree 2 poles (7.1713, 11.3777) (7.1374, 11.3425) (7.0521, 11.306) (7.0009, 11.306) knots 0 0 0 1 2 2 2
  spline S141 degree 2 poles (7.0009, 11.306) (6.9496, 11.306) (6.865, 11.3406) (6.8329, 11.3752) knots 0 0 0 1 2 2 2
  spline S142 degree 2 poles (6.8329, 11.3752) (6.7934, 11.4166) (6.7489, 11.5555) (6.7489, 11.6568) knots 0 0 0 1 2 2 2
  spline S143 degree 2 poles (6.7489, 11.6568) (6.7489, 11.7562) (6.7897, 11.9161) (6.8323, 11.9754) knots 0 0 0 1 2 2 2
  spline S144 degree 2 poles (6.8323, 11.9754) (6.8737, 12.0335) (7.0046, 12.0983) (7.0904, 12.0983) knots 0 0 0 1 2 2 2
  spline S145 degree 2 poles (7.0904, 12.0983) (7.1157, 12.0983) (7.1602, 12.0934) (7.1769, 12.0878) knots 0 0 0 1 2 2 2
  line L132 (7.1769, 12.0878) -> (7.1769, 11.9896)
  line L133 (7.1769, 11.9896) -> (7.1725, 11.9896)
  spline S146 degree 2 poles (7.1725, 11.9896) (7.1583, 11.997) (7.1065, 12.01) (7.0768, 12.01) knots 0 0 0 1 2 2 2
  spline S147 degree 2 poles (7.0768, 12.01) (6.9817, 12.01) (6.865, 11.8816) (6.8539, 11.7556) knots 0 0 0 1 2 2 2
  spline S148 degree 2 poles (6.8539, 11.7556) (6.8903, 11.7809) (6.9669, 11.8087) (7.0126, 11.8087) knots 0 0 0 1 2 2 2
  spline S149 degree 2 poles (7.0126, 11.8087) (7.0571, 11.8087) (7.1238, 11.7908) (7.1602, 11.7636) knots 0 0 0 1 2 2 2
  spline S150 degree 2 poles (7.1602, 11.7636) (7.2022, 11.7321) (7.2429, 11.6346) (7.2429, 11.5691) knots 0 0 0 1 2 2 2
  spline S151 degree 2 poles (7.1392, 11.5648) (7.1392, 11.6117) (7.1145, 11.6753) (7.0873, 11.6975) knots 0 0 0 1 2 2 2
  spline S152 degree 2 poles (7.0873, 11.6975) (7.067, 11.7136) (7.0163, 11.7241) (6.9898, 11.7241) knots 0 0 0 1 2 2 2
  spline S153 degree 2 poles (6.9898, 11.7241) (6.954, 11.7241) (6.8866, 11.7025) (6.8539, 11.6821) knots 0 0 0 1 2 2 2
  spline S154 degree 2 poles (6.8539, 11.6821) (6.8533, 11.671) (6.8521, 11.65) (6.8521, 11.6339) knots 0 0 0 1 2 2 2
  spline S155 degree 2 poles (6.8521, 11.6339) (6.8521, 11.5549) (6.8829, 11.458) (6.9064, 11.4326) knots 0 0 0 1 2 2 2
  spline S156 degree 2 poles (6.9064, 11.4326) (6.928, 11.4086) (6.9749, 11.3894) (7.0015, 11.3894) knots 0 0 0 1 2 2 2
  spline S157 degree 2 poles (7.0015, 11.3894) (7.0633, 11.3894) (7.1392, 11.4771) (7.1392, 11.5648) knots 0 0 0 1 2 2 2
  line L134 (7.8117, 11.9699) -> (7.4819, 11.3221)
  line L135 (7.4819, 11.3221) -> (7.3732, 11.3221)
  line L136 (7.3732, 11.3221) -> (7.7215, 11.9946)
  line L137 (7.7215, 11.9946) -> (7.3282, 11.9946)
  line L138 (7.3282, 11.9946) -> (7.3282, 12.0841)
  line L139 (7.3282, 12.0841) -> (7.8117, 12.0841)
  line L140 (7.8117, 12.0841) -> (7.8117, 11.9699)
  spline S158 degree 2 poles (8.3792, 11.7031) (8.3792, 11.4981) (8.26, 11.306) (8.1359, 11.306) knots 0 0 0 1 2 2 2
  spline S159 degree 2 poles (8.1359, 11.306) (8.0099, 11.306) (7.8919, 11.5018) (7.8919, 11.7025) knots 0 0 0 1 2 2 2
  spline S160 degree 2 poles (7.8919, 11.7025) (7.8919, 11.9087) (8.0111, 12.0995) (8.1359, 12.0995) knots 0 0 0 1 2 2 2
  spline S161 degree 2 poles (8.1359, 12.0995) (8.2612, 12.0995) (8.3792, 11.9019) (8.3792, 11.7031) knots 0 0 0 1 2 2 2
  spline S162 degree 2 poles (8.2482, 11.4709) (8.2631, 11.5086) (8.2754, 11.6247) (8.2754, 11.7031) knots 0 0 0 1 2 2 2
  spline S163 degree 2 poles (8.2754, 11.7031) (8.2754, 11.7815) (8.2631, 11.897) (8.2476, 11.9359) knots 0 0 0 1 2 2 2
  spline S164 degree 2 poles (8.2476, 11.9359) (8.2322, 11.9748) (8.1785, 12.0149) (8.1359, 12.0149) knots 0 0 0 1 2 2 2
  spline S165 degree 2 poles (8.1359, 12.0149) (8.0932, 12.0149) (8.0383, 11.9748) (8.0222, 11.9347) knots 0 0 0 1 2 2 2
  spline S166 degree 2 poles (8.0222, 11.9347) (8.0068, 11.8958) (7.9957, 11.7772) (7.9957, 11.7025) knots 0 0 0 1 2 2 2
  spline S167 degree 2 poles (7.9957, 11.7025) (7.9957, 11.6222) (8.0056, 11.5148) (8.0216, 11.4728) knots 0 0 0 1 2 2 2
  spline S168 degree 2 poles (8.0216, 11.4728) (8.0364, 11.4333) (8.0914, 11.3906) (8.1359, 11.3906) knots 0 0 0 1 2 2 2
  spline S169 degree 2 poles (8.1359, 11.3906) (8.1778, 11.3906) (8.2328, 11.4308) (8.2482, 11.4709) knots 0 0 0 1 2 2 2
  line L141 (8.9084, 11.3221) -> (8.5366, 11.3221)
  line L142 (8.5366, 11.3221) -> (8.5366, 11.3999)
  line L143 (8.5366, 11.3999) -> (8.6749, 11.3999)
  line L144 (8.6749, 11.3999) -> (8.6749, 11.9106)
  line L145 (8.6749, 11.9106) -> (8.5366, 11.9106)
  line L146 (8.5366, 11.9106) -> (8.5366, 11.9804)
  spline S170 degree 2 poles (8.5366, 11.9804) (8.615, 11.9804) (8.6891, 12.0248) (8.6941, 12.0866) knots 0 0 0 1 2 2 2
  line L147 (8.6941, 12.0866) -> (8.7731, 12.0866)
  line L148 (8.7731, 12.0866) -> (8.7731, 11.3999)
  line L149 (8.7731, 11.3999) -> (8.9084, 11.3999)
  line L150 (8.9084, 11.3999) -> (8.9084, 11.3221)
  line L151 (1.6731, 10.0675) -> (1.5767, 10.0675)
  line L152 (1.5767, 10.0675) -> (1.5767, 10.1255)
  spline S171 degree 2 poles (1.5767, 10.1255) (1.5545, 10.107) (1.5218, 10.0823) (1.4995, 10.0718) knots 0 0 0 1 2 2 2
  spline S172 degree 2 poles (1.4995, 10.0718) (1.4792, 10.0619) (1.4353, 10.0514) (1.4063, 10.0514) knots 0 0 0 1 2 2 2
  spline S173 degree 2 poles (1.4063, 10.0514) (1.3594, 10.0514) (1.2803, 10.0903) (1.2525, 10.128) knots 0 0 0 1 2 2 2
  spline S174 degree 2 poles (1.2525, 10.128) (1.2247, 10.1657) (1.1939, 10.2768) (1.1939, 10.3491) knots 0 0 0 1 2 2 2
  spline S175 degree 2 poles (1.1939, 10.3491) (1.1939, 10.4244) (1.2328, 10.5343) (1.2667, 10.5757) knots 0 0 0 1 2 2 2
  spline S176 degree 2 poles (1.2667, 10.5757) (1.2982, 10.6127) (1.3865, 10.6554) (1.4353, 10.6554) knots 0 0 0 1 2 2 2
  spline S177 degree 2 poles (1.4353, 10.6554) (1.4779, 10.6554) (1.5415, 10.6362) (1.5767, 10.6164) knots 0 0 0 1 2 2 2
  line L153 (1.5767, 10.6164) -> (1.5767, 10.8635)
  line L154 (1.5767, 10.8635) -> (1.6731, 10.8635)
  line L155 (1.6731, 10.8635) -> (1.6731, 10.0675)
  line L156 (1.5767, 10.2064) -> (1.5767, 10.5368)
  spline S178 degree 2 poles (1.5767, 10.5368) (1.5409, 10.5541) (1.4841, 10.567) (1.4514, 10.567) knots 0 0 0 1 2 2 2
  spline S179 degree 2 poles (1.4514, 10.567) (1.3773, 10.567) (1.2933, 10.4559) (1.2933, 10.3509) knots 0 0 0 1 2 2 2
  spline S180 degree 2 poles (1.2933, 10.3509) (1.2933, 10.2497) (1.3575, 10.1428) (1.4285, 10.1428) knots 0 0 0 1 2 2 2
  spline S181 degree 2 poles (1.4285, 10.1428) (1.4662, 10.1428) (1.5428, 10.1774) (1.5767, 10.2064) knots 0 0 0 1 2 2 2
  spline S182 degree 2 poles (2.1312, 10.128) (2.1195, 10.1194) (2.08, 10.0885) (2.0615, 10.0792) knots 0 0 0 1 2 2 2
  spline S183 degree 2 poles (2.0615, 10.0792) (2.0361, 10.0656) (1.9886, 10.0514) (1.9454, 10.0514) knots 0 0 0 1 2 2 2
  spline S184 degree 2 poles (1.9454, 10.0514) (1.9102, 10.0514) (1.8466, 10.078) (1.8225, 10.1021) knots 0 0 0 1 2 2 2
  spline S185 degree 2 poles (1.8225, 10.1021) (1.7996, 10.1255) (1.7719, 10.1947) (1.7719, 10.233) knots 0 0 0 1 2 2 2
  spline S186 degree 2 poles (1.7719, 10.233) (1.7719, 10.2923) (1.8219, 10.3762) (1.8762, 10.4003) knots 0 0 0 1 2 2 2
  spline S187 degree 2 poles (1.8762, 10.4003) (1.9244, 10.4226) (2.0553, 10.4392) (2.1312, 10.4435) knots 0 0 0 1 2 2 2
  line L157 (2.1312, 10.4435) -> (2.1312, 10.4621)
  spline S188 degree 2 poles (2.1312, 10.4621) (2.1312, 10.4954) (2.1109, 10.5368) (2.0923, 10.5485) knots 0 0 0 1 2 2 2
  spline S189 degree 2 poles (2.0923, 10.5485) (2.0738, 10.5603) (2.0207, 10.5677) (1.9923, 10.5677) knots 0 0 0 1 2 2 2
  spline S190 degree 2 poles (1.9923, 10.5677) (1.959, 10.5677) (1.8688, 10.5479) (1.8237, 10.5288) knots 0 0 0 1 2 2 2
  line L158 (1.8237, 10.5288) -> (1.8182, 10.5288)
  line L159 (1.8182, 10.5288) -> (1.8182, 10.6269)
  spline S191 degree 2 poles (1.8182, 10.6269) (1.8447, 10.6344) (1.9441, 10.6529) (1.9929, 10.6529) knots 0 0 0 1 2 2 2
  spline S192 degree 2 poles (1.9929, 10.6529) (2.0522, 10.6529) (2.1331, 10.6344) (2.1652, 10.6103) knots 0 0 0 1 2 2 2
  spline S193 degree 2 poles (2.1652, 10.6103) (2.1967, 10.5868) (2.2276, 10.5121) (2.2276, 10.4584) knots 0 0 0 1 2 2 2
  line L160 (2.2276, 10.4584) -> (2.2276, 10.0675)
  line L161 (2.2276, 10.0675) -> (2.1312, 10.0675)
  line L162 (2.1312, 10.0675) -> (2.1312, 10.128)
  line L163 (2.1312, 10.2083) -> (2.1312, 10.367)
  spline S194 degree 2 poles (2.1312, 10.367) (2.0967, 10.3639) (1.9923, 10.3534) (1.9596, 10.3435) knots 0 0 0 1 2 2 2
  spline S195 degree 2 poles (1.9596, 10.3435) (1.9213, 10.3318) (1.8713, 10.283) (1.8713, 10.2398) knots 0 0 0 1 2 2 2
  spline S196 degree 2 poles (1.8713, 10.2398) (1.8713, 10.1904) (1.9269, 10.1404) (1.98, 10.1404) knots 0 0 0 1 2 2 2
  spline S197 degree 2 poles (1.98, 10.1404) (2.025, 10.1404) (2.0991, 10.1793) (2.1312, 10.2083) knots 0 0 0 1 2 2 2
  line L164 (2.666, 10.5362) -> (2.6611, 10.5362)
  spline S198 degree 2 poles (2.6611, 10.5362) (2.6499, 10.5393) (2.6259, 10.5405) (2.6092, 10.5405) knots 0 0 0 1 2 2 2
  spline S199 degree 2 poles (2.6092, 10.5405) (2.5703, 10.5405) (2.4937, 10.5065) (2.4591, 10.4732) knots 0 0 0 1 2 2 2
  line L165 (2.4591, 10.4732) -> (2.4591, 10.0675)
  line L166 (2.4591, 10.0675) -> (2.3628, 10.0675)
  line L167 (2.3628, 10.0675) -> (2.3628, 10.6393)
  line L168 (2.3628, 10.6393) -> (2.4591, 10.6393)
  line L169 (2.4591, 10.6393) -> (2.4591, 10.5541)
  spline S200 degree 2 poles (2.4591, 10.5541) (2.5116, 10.601) (2.5901, 10.6393) (2.6271, 10.6393) knots 0 0 0 1 2 2 2
  spline S201 degree 2 poles (2.6271, 10.6393) (2.6419, 10.6393) (2.6567, 10.6381) (2.666, 10.6362) knots 0 0 0 1 2 2 2
  line L170 (2.666, 10.6362) -> (2.666, 10.5362)
  spline S202 degree 2 poles (2.8951, 10.0539) (2.8377, 10.0539) (2.7383, 10.0848) (2.7055, 10.1021) knots 0 0 0 1 2 2 2
  line L171 (2.7055, 10.1021) -> (2.7055, 10.2101)
  line L172 (2.7055, 10.2101) -> (2.7105, 10.2101)
  spline S203 degree 2 poles (2.7105, 10.2101) (2.7228, 10.2003) (2.7562, 10.1768) (2.7839, 10.1638) knots 0 0 0 1 2 2 2
  spline S204 degree 2 poles (2.7839, 10.1638) (2.808, 10.1521) (2.8673, 10.1348) (2.8988, 10.1348) knots 0 0 0 1 2 2 2
  spline S205 degree 2 poles (2.8988, 10.1348) (2.9217, 10.1348) (2.9741, 10.1453) (2.9865, 10.1539) knots 0 0 0 1 2 2 2
  spline S206 degree 2 poles (2.9865, 10.1539) (3.0044, 10.1657) (3.0205, 10.1922) (3.0205, 10.2194) knots 0 0 0 1 2 2 2
  spline S207 degree 2 poles (3.0205, 10.2194) (3.0205, 10.2534) (2.9834, 10.2886) (2.9359, 10.3003) knots 0 0 0 1 2 2 2
  spline S208 degree 2 poles (2.9359, 10.3003) (2.9173, 10.3046) (2.858, 10.317) (2.8327, 10.3238) knots 0 0 0 1 2 2 2
  spline S209 degree 2 poles (2.8327, 10.3238) (2.7673, 10.3429) (2.708, 10.4219) (2.708, 10.4781) knots 0 0 0 1 2 2 2
  spline S210 degree 2 poles (2.708, 10.4781) (2.708, 10.5559) (2.8247, 10.6529) (2.921, 10.6529) knots 0 0 0 1 2 2 2
  spline S211 degree 2 poles (2.921, 10.6529) (2.9686, 10.6529) (3.0649, 10.6294) (3.0976, 10.6115) knots 0 0 0 1 2 2 2
  line L173 (3.0976, 10.6115) -> (3.0976, 10.5084)
  line L174 (3.0976, 10.5084) -> (3.0927, 10.5084)